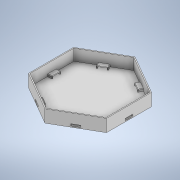
# Autodesk Inventor part: hexlight
Saved by Autodesk Inventor 2020 (Build 240168000, 168)
## iProperties
Created: 2019-09-25
Part Number: hexlight
Material: Generic
Document SubType Name: Modeling
Designer: Adam
Density: 1 g/cm^3
Appearance: Default
Author: Adam
Autodesk Inventor part; units mm, degrees
ref_plane "YZ Plane" through (0, 0, 0) normal (1, 0, 0) x (0, 1, 0)
ref_plane "XZ Plane" through (0, 0, 0) normal (0, 1, 0) x (-1, 0, 0)
ref_plane "XY Plane" through (0, 0, 0) normal (0, 0, 1) x (1, 0, 0)
sketch "Sketch1" plane through (0, 0, 0) normal (0, 1, 0) x (-1, 0, 0)
  line L0 (69.282032, -40) -> (0, -80)
  line L1 (0, -80) -> (-69.282032, -40)
  line L2 (-69.282032, -40) -> (-69.282032, 40)
  line L3 (-69.282032, 40) -> (0, 80)
  line L4 (0, 80) -> (69.282032, 40)
  line L5 (69.282032, 40) -> (69.282032, -40)
  point P0 (0, 0)
  point P1 (0, 0)
  dimension "d1" = 80
  dimension "d2" = 0
  constraints: 12 end point, 1 coincident, 13 other
  measures "d1" distance of L4.end L0.start
  measures "d2" horizontal distance of point (0, 0) L0.end
extrude "Extrusion1" add sketch "Sketch1" along normal blind 22
sketch "Sketch2" plane through (0, 22, 0) normal (0, 1, 0) x (1, 0, 0)
  line L0 (0, 78) -> (67.549981, 39)
  line L1 (67.549981, 39) -> (67.549981, -39)
  line L2 (67.549981, -39) -> (0, -78)
  line L3 (0, -78) -> (-67.549981, -39)
  line L4 (-67.549981, -39) -> (-67.549981, 39)
  line L5 (-67.549981, 39) -> (0, 78)
  point P0 (0, 0)
  point P1 (0, 0)
  dimension "d5" = 0
  dimension "d6" = 78
  constraints: 12 end point, 1 coincident, 13 other
  measures "d5" horizontal distance of point (0, 0) L0.start
  measures "d6" distance of L3.end L4.end
extrude "Extrusion2" cut sketch "Sketch2" against normal blind 20
sketch "Sketch4" plane through (67.549981, 22, -39) normal (-1, 0, 0) x (0, 0, 1)
  line L0 (0, -20) -> (78, -20) projected
  line L1 (32.5, -20) -> (45.5, -20)
  line L2 (45.5, -20) -> (45.5, -16.75)
  line L3 (45.5, -16.75) -> (32.5, -16.75)
  line L4 (32.5, -16.75) -> (32.5, -20)
  line L5 (-1, -22) -> (-1, 0) projected
  point P0 (39, -22)
  dimension "d9" = 13
  dimension "d10" = 3.25
  dimension "d11" = 33.5
  constraints: 8 end point, 2 parallel, 1 horizontal, 1 perpendicular, 1 point on line
  measures "d9" distance of L2.end L3.end
  measures "d10" distance of L1.end L2.end
  measures "d11" distance between parallel lines of L5 L4
sketch "Sketch5" plane through (0, 2, 0) normal (0, 1, 0) x (1, 0, 0)
  line L0 (67.549981, 39) -> (67.549981, -39)
  line L1 (59.549981, -8) -> (67.549981, -8)
  line L2 (67.549981, -8) -> (67.549981, 8)
  line L3 (67.549981, 8) -> (59.549981, 8)
  line L4 (59.549981, 8) -> (59.549981, -8)
  point P0 (0, 0)
  point P1 (69.282032, 40)
  dimension "d12" = 16
  dimension "d13" = 8
  dimension "d14" = 32
  constraints: 8 end point, 2 parallel, 1 horizontal, 1 perpendicular, 1 point on line
  measures "d12" distance of L3.end L1.start
  measures "d13" distance of L2.end L3.end
  measures "d14" distance from line of point (69.282, 40) L3
extrude "Extrusion3" add sketch "Sketch5" along normal blind 4
extrude "Extrusion4" cut sketch "Sketch4" along normal mid plane 16
fillet "Fillet1" radius 1 5 edges at (63.55, 6, -8) (59.55, 4, -8) (59.55, 6, 0) (59.55, 4, 8) (63.55, 6, 8)
pattern_circular "Circular Pattern1" count 6 over 360 about axis through (0, -10, 0) along (0, 1, 0) of "Fillet1", "Extrusion3", "Extrusion4"
body "Solid1"
